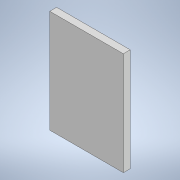
# Autodesk Inventor part: acrylicwindow
Saved by Autodesk Inventor 2022.2 (Build 262287030, 287C)
## iProperties
Created: 2022-03-16
Part Number: acrylicwindow
Material: Generic
Document SubType Name: Modeling
Designer: Tapendra
Density: 1 g/cm^3
Appearance: Default
Author: Tapendra
Autodesk Inventor part; units mm, degrees
ref_plane "YZ Plane" through (0, 0, 0) normal (1, 0, 0) x (0, 1, 0)
ref_plane "XZ Plane" through (0, 0, 0) normal (0, 1, 0) x (-1, 0, 0)
ref_plane "XY Plane" through (0, 0, 0) normal (0, 0, 1) x (1, 0, 0)
sketch "Sketch1" plane through (0, 0, 0) normal (0, 0, 1) x (1, 0, 0)
  line L0 (-37.5, 52.5) -> (37.5, 52.5)
  line L1 (37.5, 52.5) -> (37.5, -52.5)
  line L2 (37.5, -52.5) -> (-37.5, -52.5)
  line L3 (-37.5, -52.5) -> (-37.5, 52.5)
  line L4 (-37.5, 52.5) -> (37.5, -52.5) construction
  line L5 (37.5, 52.5) -> (-37.5, -52.5) construction
  point P0 (0, 0)
  dimension "d0" = 75
  dimension "d1" = 105
  constraints: 12 end point, 2 midpoint, 2 parallel, 1 horizontal, 1 perpendicular
  measures "d0" distance of L0.start L0.end
  measures "d1" distance of L0.end L1.end
extrude "Extrusion1" add sketch "Sketch1" along normal mid plane 7
body "Solid1"
